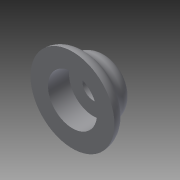
# Autodesk Inventor part: galka enkodera
Saved by Autodesk Inventor 2014 (Build 180170000, 170)
## iProperties
Created: 2018-04-02
Part Number: galka enkodera
Material: Generic
Document SubType Name: Modeling
Designer: HP820
Density: 1 g/cm^3
Appearance: Default
Author: HP820
Autodesk Inventor part; units mm, degrees
ref_plane "YZ Plane" through (0, 0, 0) normal (1, 0, 0) x (0, 1, 0)
ref_plane "XZ Plane" through (0, 0, 0) normal (0, 1, 0) x (-1, 0, 0)
ref_plane "XY Plane" through (0, 0, 0) normal (0, 0, 1) x (1, 0, 0)
sketch "Sketch1" plane through (0, 0, 0) normal (0, 1, 0) x (-1, 0, 0)
  arc A0 (-2.05, -2.3917) -> (-2.05, 2.3917) centre (0, 0) ccw
  line L0 (3.15, 0) -> (-2.05, 0)
  line L1 (-2.05, 0) -> (-2.05, -2.3917)
  line L2 (-2.05, 0) -> (-2.05, 2.3917)
  circle A1 centre (0, 0) radius 8
  dimension "d0" = 6.3
  dimension "d1" = 5.2
  dimension "d2" = 16
  constraints: 6 end point, 3 point on circle, 2 centre point, 2 coincident, 1 collinear, 1 horizontal, 1 perpendicular
  measures "d0" diameter of A0
  measures "d1" distance of L0.start L0.end
  measures "d2" diameter of A1
extrude "Extrusion1" add sketch "Sketch1" along normal blind 10
sketch "Sketch2" plane through (0, 10, 0) normal (0, 1, 0) x (1, 0, 0)
  arc A0 (2.05, 2.3917) -> (2.05, -2.3917) centre (0, 0) ccw projected
  line L0 (2.05, 2.3917) -> (2.05, -2.3917) projected
extrude "Extrusion2" add sketch "Sketch2" against normal blind 1
sketch "Sketch3" plane through (0, 0, 0) normal (0, -1, 0) x (1, 0, 0)
  arc A0 (2.05, 2.3917) -> (2.05, -2.3917) centre (0, 0) ccw projected
  line L0 (2.05, 2.3917) -> (2.05, -2.3917) projected
  circle A1 centre (0, 0) radius 7
  dimension "d7" = 14
  constraints: 1 centre point, 1 coincident
  measures "d7" diameter of A1
extrude "Extrusion3" cut sketch "Sketch3" against normal blind 6
sketch "Sketch4" plane through (0, 0, 0) normal (0, -1, 0) x (1, 0, 0)
  circle A0 centre (0, 0) radius 8 projected
  circle A1 centre (0, 0) radius 12
  dimension "d10" = 24
  constraints: 1 centre point, 1 coincident
  measures "d10" diameter of A1
extrude "Extrusion4" add sketch "Sketch4" against normal blind 3
fillet "Fillet1" radius 4 3 edges at (8, 3, 0) (-12, 3, 0) (8, 10, 0)
body "Solid1"
